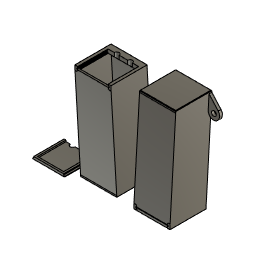
MAX31820WeatherStation (Autodesk Fusion 360 design; units mm, degrees)
Autodesk Fusion 360 part; units mm, degrees
sketch "case base" plane through (0, 0, 0) normal (0, 0, 1) x (1, 0, 0)
  line L0 (-17, 17) -> (17, 17)
  line L1 (17, 17) -> (17, -17)
  line L2 (17, -17) -> (-17, -17)
  line L3 (-17, -17) -> (-17, 17)
  line L4 (-17, 17) -> (17, -17) construction
  line L5 (17, 17) -> (-17, -17) construction
  line L6 (-19, 19) -> (19, 19)
  line L7 (19, 19) -> (19, -19)
  line L8 (19, -19) -> (-19, -19)
  line L9 (-19, -19) -> (-19, 19)
  line L10 (-19, 19) -> (19, -19) construction
  line L11 (19, 19) -> (-19, -19) construction
  dimension "d1" = 34
  dimension "d2" = 2
  dimension "d3" = 2
  constraint perpendicular L0 L1
  constraint parallel L0 L2
  constraint parallel L1 L3
  constraint horizontal L0
  constraint coincident L4 origin
  constraint coincident L5 origin
  constraint perpendicular L6 L7
  constraint parallel L6 L8
  constraint parallel L7 L9
  constraint horizontal L6
  constraint coincident L10 origin
  constraint coincident L11 origin
  constraint equal L1 L2
  measures "d1" distance of L0.start L0.end
  measures "d2" horizontal distance of L0.start L6.start
  measures "d3" vertical distance of L0.start L6.start
ref_plane "WorkPlane1" through (0, 0, 100) normal (0, 0, 1) x (1, 0, 0)
sketch "case top" plane through (0, 0, 100) normal (0, 0, 1) x (1, 0, 0)
  line L0 (-17, 23) -> (17, 23)
  line L1 (17, 23) -> (17, -11)
  line L2 (17, -11) -> (-17, -11)
  line L3 (-17, -11) -> (-17, 23)
  line L4 (-19, 25) -> (19, 25)
  line L5 (19, 25) -> (19, -13)
  line L6 (19, -13) -> (-19, -13)
  line L7 (-19, -13) -> (-19, 25)
  line L8 (-17, 23) -> (17, -11) construction
  point P0 (0, 6)
  dimension "d5" = 34
  dimension "d6" = 2
  dimension "d7" = 2
  dimension "d8" = 2
  dimension "d9" = 2
  dimension "d12" = 6
  constraint horizontal L0
  constraint vertical L1
  constraint horizontal L2
  constraint vertical L3
  constraint equal L0 L3
  constraint horizontal L4
  constraint vertical L5
  constraint horizontal L6
  constraint vertical L7
  constraint midpoint L8 P0
  constraint vertical origin P0
  measures "d5" distance of L0.start L0.end
  measures "d6" horizontal distance of L0.start L4.start
  measures "d7" vertical distance of L0.start L4.start
  measures "d8" horizontal distance of L1.end L5.end
  measures "d9" vertical distance of L1.end L5.end
  measures "d12" distance of origin P0
loft "Loft1" add profiles "case base", "case top" section 1 contours L0 L1 L2 L3 | L6 L7 L8 L9 section 2 contours L0 L1 L2 L3 | L4 L5 L6 L7 makes body 1
loft "Loft2" cut profiles "case base", "case top" section 1 contours L0 L1 L2 L3 section 2 contours L0 L1 L2 L3 bodies 1
extrude "Extrude1" add sketch "case top" along normal blind 2 contours L0 L1 L2 L3 | L4 L5 L6 L7 bodies 1
sketch "nail loop" plane through (0, 18.9318, -1.1359) normal (0, 0.998205, -0.059892) x (-1, 0, 0)
  line L0 (-19, 1.138) -> (19, 1.138)
  line L1 (19, 1.138) -> (19, 101.3178)
  line L2 (19, 101.3178) -> (-19, 101.3178)
  line L3 (-19, 101.3178) -> (-19, 1.138)
  line L4 (-29.2426, 91.0752) -> (-19, 101.3178)
  line L5 (-19, 101.3178) -> (-19, 86.8325)
  arc A0 (-29.2426, 91.0752) -> (-19, 86.8325) centre (-25, 86.8325) ccw
  circle A1 centre (-25, 86.8325) radius 2.5
  dimension "d15" = 45
  dimension "d16" = 6
  dimension "d17" = 5
  constraint vertical L5
  constraint coincident L4.start A0.start
  constraint tangent L4 A0
  constraint coincident L5.end A0.end
  constraint tangent L5 A0
  constraint coincident A0.centre A1.centre
  constraint coincident L2.end L3.start
  measures "d15" angle of L4 L5
  measures "d16" radius of A0
  measures "d17" diameter of A1
extrude "Extrude3" add sketch "nail loop" against normal blind 3 separate body contours L3 L4 L5 A0 makes body 2
mirror "Mirror1" about plane through (0, 0, 0) normal (1, 0, 0) of bodies 2 makes body 3
combine "Combine1" operation add target body 1 tool bodies 2 3
sketch "case bottom back" plane through (0, 0, 0) normal (1, 0, 0) x (0, 1, 0)
  line L0 (19, -3) -> (19, 7)
  line L1 (19, 7) -> (13, 1)
  line L2 (13, 1) -> (13, -3)
  line L3 (13, -3) -> (19, -3)
  point P0 (19, 0)
  dimension "d77" = 45
  dimension "d78" = 4
  dimension "d79" = 6
  dimension "d91" = 3
  constraint vertical L0
  constraint perpendicular L0 L3
  constraint perpendicular L2 L3
  constraint vertical L0.start P0
  measures "d77" angle of L0 L1
  measures "d78" distance of L1.end L2.end
  measures "d79" distance of L0.start L2.end
  measures "d91" distance of L0.start P0
extrude "Extrude10" add sketch "case bottom back" along normal mid plane 38 separate body makes body 4
sketch "one rail" plane through (0, 0, 0) normal (0, 1, 0) x (1, 0, 0)
  line L0 (19, -2) -> (17, -2)
  line L1 (17, -2) -> (16, -1)
  line L2 (16, -1) -> (16, 0)
  line L3 (16, 0) -> (17, 0)
  line L4 (17, 0) -> (17, 1)
  line L5 (17, 1) -> (16, 2)
  line L6 (16, 2) -> (16, 3)
  line L7 (16, 3) -> (19, 3)
  line L8 (19, 3) -> (19, -2)
  point P0 (19, 3)
  dimension "d82" = 135
  dimension "d83" = 135
  dimension "d84" = 1
  dimension "d85" = 1
  dimension "d86" = 1
  dimension "d87" = 1
  dimension "d89" = 1
  dimension "d90" = 2
  constraint horizontal L0
  constraint perpendicular L2 L3
  constraint perpendicular L0 L8
  constraint perpendicular L7 L8
  constraint perpendicular L6 L7
  constraint perpendicular L3 L4
  constraint parallel L2 L8
  constraint vertical L2.end L5.end
  constraint coincident P0 L7.end
  measures "d82" angle of L5 L6
  measures "d83" angle of L1 L2
  measures "d84" distance of L5.end L6.end
  measures "d85" vertical distance of L4.end L5.end
  measures "d86" distance of L3.end L4.end
  measures "d87" vertical distance of L0.end L1.end
  measures "d89" distance of L1.end L2.end
  measures "d90" distance of L0.start L0.end
extrude "Extrude11" add sketch "one rail" along normal mid plane 38 separate body makes body 5
mirror "Mirror3" about plane through (0, 0, 0) normal (1, 0, 0) of bodies 5 makes body 6
combine "Combine2" operation add target body 1 tool bodies 4 5 6
sketch "cap" plane through (0, 0, 0) normal (0, 1, 0) x (1, 0, 0)
  line L0 (16.75, 0) -> (-16.75, 0)
  line L1 (-16.75, 0) -> (-16.75, 1)
  line L2 (-16.75, 1) -> (-15.75, 2)
  line L3 (-15.75, 2) -> (-15.75, 3)
  line L4 (-15.75, 3) -> (15.75, 3)
  line L5 (15.75, 3) -> (15.75, 2)
  line L6 (15.75, 2) -> (16.75, 1)
  line L7 (16.75, 1) -> (16.75, 0)
  point P0 (0, 3)
  dimension "d95" = 135
  dimension "d96" = 135
  dimension "d97" = 1
  dimension "d98" = 1
  dimension "d99" = 1
  dimension "d102" = 33.5
  constraint horizontal L0
  constraint perpendicular L0 L1
  constraint perpendicular L3 L4
  constraint perpendicular L4 L5
  constraint perpendicular L0 L7
  constraint midpoint L4 P0
  constraint parallel L0 L4
  constraint equal L3 L5
  constraint equal L2 L6
  constraint vertical origin P0
  constraint horizontal origin L0.start
  measures "d95" angle of L2 L3
  measures "d96" angle of L5 L6
  measures "d97" distance of L0.end L1.end
  measures "d98" vertical distance of L1.end L2.end
  measures "d99" vertical distance of L2.end L3.end
  measures "d102" distance of L0.start L0.end
extrude "Extrude12" add sketch "cap" along normal blind 13 and the other way blind 19 separate body makes body 7
sketch "cap inset" plane through (0, 0, -3) normal (0, 0, -1) x (1, 0, 0)
  line L0 (-15.75, 19) -> (-15.75, -13)
  line L1 (-15.75, -13) -> (15.75, -13)
  line L2 (15.75, -13) -> (15.75, 19)
  line L3 (15.75, 19) -> (-15.75, 19)
  line L4 (-13.75, 17) -> (13.75, 17)
  line L5 (13.75, 17) -> (13.75, -13)
  line L6 (13.75, -13) -> (-13.75, -13)
  line L7 (-13.75, -13) -> (-13.75, 17)
  dimension "d107" = 2
  dimension "d110" = 2
  dimension "d111" = 2
  constraint horizontal L4
  constraint vertical L5
  constraint horizontal L6
  constraint vertical L7
  constraint horizontal L1.end L5.end
  measures "d107" horizontal distance of L0.start L4.start
  measures "d110" horizontal distance of L1.end L5.end
  measures "d111" vertical distance of L0.start L4.start
extrude "Extrude13" cut sketch "cap inset" against normal blind 1.5 contours L1 L4 L5 L6 L7 bodies 7
sketch "one cutting rod" plane through (0, 0, 0) normal (0, 0, 1) x (1, 0, 0)
  circle A0 centre (-7, 13) radius 2.5
  dimension "d116" = 5
  dimension "d117" = 13
  dimension "d118" = 7
  measures "d116" diameter of A0
  measures "d117" vertical distance of origin A0.centre
  measures "d118" horizontal distance of origin A0.centre
extrude "Extrude14" add sketch "one cutting rod" along normal mid plane 20 separate body makes body 8
mirror "Mirror4" about plane through (0, 0, 0) normal (1, 0, 0) of bodies 8 makes body 9
combine "Combine3" operation cut target body 7 tool bodies 8 9 keep tools
combine "Combine4" operation cut target body 1 tool bodies 8 9
chamfer "Chamfer1" distance 0.5 angle 45 4 edges at (0, 25, 102) (-19, 6, 102) (0, -13, 102) (19, 6, 102) on bodies 1
chamfer "Chamfer2" distance 0.5 angle 45 8 edges at (16.75, -3, 0) (0, -19, 0) (-16.75, -3, 0) (-13.125, 13, 0) (-7, 10.5, 0) (0, 13, 0) (7, 10.5, 0) (13.125, 13, 0) on bodies 7
copy_body "CopyPasteBodies1" bodies 1 makes body 10
move_body "Move1" bodies 10 to x (-1, 0, 0) y (0, 1, 0) z (0, 0, -1) at (-62, 0, 94)
copy_body "CopyPasteBodies2" bodies 7 makes body 11
move_body "Move2" bodies 11 to x (-1, 0, 0) y (0, 1, 0) z (0, 0, -1) at (-108.5, 0, -11)
named bodies: "case", "right nail loop", "left nail loop", "case bottom back", "right case rail", "left case rail", "cap", "left cutting rod", "right cutting rod", "case for printing", "cap for printing"
